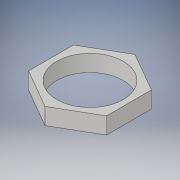
# Autodesk Inventor part: Strom_Mutter
Saved by Autodesk Inventor 2019 (Build 230136000, 136)
## iProperties
Created: 2020-06-15
Part Number: Strom_Mutter
Material: Generic
Document SubType Name: Modeling
Designer: Erle
Density: 1 g/cm^3
Appearance: Default
Author: Erle
Autodesk Inventor part; units mm, degrees
ref_plane "YZ Plane" through (0, 0, 0) normal (1, 0, 0) x (0, 1, 0)
ref_plane "XZ Plane" through (0, 0, 0) normal (0, 1, 0) x (-1, 0, 0)
ref_plane "XY Plane" through (0, 0, 0) normal (0, 0, 1) x (1, 0, 0)
sketch "Sketch1" plane through (0, 0, 0) normal (0, 1, 0) x (-1, 0, 0)
  circle A0 centre (0, 0) radius 4
  line L0 (0, -5.4271) -> (-4.7, -2.7135)
  line L1 (-4.7, -2.7135) -> (-4.7, 2.7135)
  line L2 (-4.7, 2.7135) -> (0, 5.4271)
  line L3 (0, 5.4271) -> (4.7, 2.7135)
  line L4 (4.7, 2.7135) -> (4.7, -2.7135)
  line L5 (4.7, -2.7135) -> (0, -5.4271)
  dimension "d0" = 8
  dimension "d1" = 9.4
  constraints: 12 end point, 2 coincident, 1 centre point, 1 vertical alignment, 13 other
  measures "d0" diameter of A0
  measures "d1" distance between parallel lines of L2 L5
extrude "Extrusion1" add sketch "Sketch1" along normal blind 2
body "Solid1"
